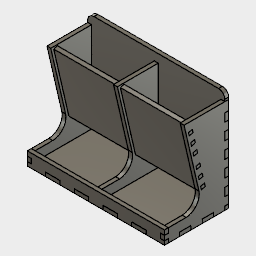
battery_box_v4 (Autodesk Fusion 360 design; units mm, degrees)
Autodesk Fusion 360 part; units mm, degrees
(part 1 of 2)
sketch "Sketch1" plane through (0, 0, 0) normal (0, 1, 0) x (1, 0, 0) in component "battery_box"
  line L0 (2.54, -2.54) -> (113.665, -2.54)
  line L1 (113.665, -2.54) -> (113.665, -54.61)
  line L2 (113.665, -54.61) -> (2.54, -54.61)
  line L3 (2.54, -54.61) -> (2.54, -2.54)
  line L4 (2.54, -2.54) -> (113.665, -2.54)
  line L5 (113.665, -2.54) -> (113.665, -5.715)
  line L6 (113.665, -5.715) -> (2.54, -5.715)
  line L7 (2.54, -5.715) -> (2.54, -2.54)
  line L8 (2.54, -2.54) -> (5.715, -2.54)
  line L9 (5.715, -2.54) -> (5.715, -54.61)
  line L10 (5.715, -54.61) -> (2.54, -54.61)
  line L11 (2.54, -54.61) -> (2.54, -2.54)
  line L12 (113.665, -2.54) -> (110.49, -2.54)
  line L13 (110.49, -2.54) -> (110.49, -54.61)
  line L14 (110.49, -54.61) -> (113.665, -54.61)
  line L15 (113.665, -54.61) -> (113.665, -2.54)
  line L16 (2.54, -54.61) -> (113.665, -54.61)
  line L17 (113.665, -54.61) -> (113.665, -51.435)
  line L18 (113.665, -51.435) -> (2.54, -51.435)
  line L19 (2.54, -51.435) -> (2.54, -54.61)
  line L20 (58.1025, -54.61) -> (56.515, -54.61)
  line L21 (56.515, -54.61) -> (56.515, -2.54) construction
  line L22 (56.515, -2.54) -> (58.1025, -2.54)
  line L23 (56.515, -2.54) -> (59.69, -2.54)
  line L24 (59.69, -2.54) -> (59.69, -54.61) construction
  line L25 (59.69, -54.61) -> (56.515, -54.61) construction
  line L26 (2.54, -20.955) -> (113.665, -20.955) construction
  line L27 (113.665, -20.955) -> (113.665, -24.13)
  line L28 (113.665, -24.13) -> (2.54, -24.13) construction
  line L29 (2.54, -24.13) -> (2.54, -20.955)
  line L30 (5.715, -5.715) -> (5.715, -2.54)
  dimension "d4" = 52.07
  dimension "d5" = 111.125
  dimension "d6" = 3.175
  dimension "d9" = 3.175
  dimension "d11" = 3.175
  dimension "d13" = 3.175
  dimension "d16" = 3.175
  dimension "d18" = 3.175
  dimension "d19" = 15.24
  measures "d4" distance of L0.start L2.end
  measures "d5" distance of L0.start L0.end
  measures "d6" distance of L0.start L6.end
  measures "d9" distance of L0.start L8.end
  measures "d11" distance of L0.end L12.end
  measures "d13" distance of L2.end L18.end
  measures "d16" distance of L21.end L23.end
  measures "d18" distance of L26.start L28.end
  measures "d19" distance of L6 L26
extrude "Extrude4" add sketch "Sketch1" against normal blind 3.175 makes body 1 in component "battery_box"
extrude "Extrude5" add sketch "Sketch1" along normal blind 7.62 separate body contours L2 L9 L13 L16 L18 L20 | L2 L3 L9 L10 L11 L16 L18 L19 | L1 L2 L13 L14 L15 L16 L17 L18 makes body 2 in component "battery_box"
extrude "Extrude6" add sketch "Sketch1" along normal blind 57.15 separate body contours L0 L3 L4 L6 L7 L8 L9 L11 L30 | L0 L4 L6 L9 L13 L22 L23 L30 | L0 L1 L4 L5 L6 L12 L13 L15 makes body 3 in component "battery_box"
extrude "Extrude7" add sketch "Sketch1" along normal blind 7.62 separate body contours L1 L6 L13 L15 L18 L27 makes body 4 in component "battery_box"
sketch "Side" plane through (113.665, 0, 0) normal (1, 0, 0) x (0, 0, -1) in component "battery_box"
  line L0 (-51.435, 0) -> (-5.715, 0)
  line L1 (-5.715, 0) -> (-5.715, 7.62)
  line L2 (-5.715, 7.62) -> (-51.435, 7.62)
  line L3 (-51.435, 7.62) -> (-51.435, 0)
  line L4 (-32.385, 45.72) -> (-5.715, 45.72)
  line L5 (-5.715, 45.72) -> (-5.715, 7.62)
  line L6 (-5.715, 7.62) -> (-20.955, 7.62)
  line L7 (-20.955, 7.62) -> (-20.955, 45.72)
  line L8 (-20.955, 45.72) -> (-5.715, 45.72)
  line L9 (-5.715, 45.72) -> (-5.715, 7.62)
  line L10 (-20.955, 7.62) -> (-24.13, 7.62)
  line L11 (-24.13, 45.72) -> (-20.955, 45.72)
  line L12 (-20.955, 45.72) -> (-20.955, 7.62)
  line L13 (-32.385, 45.72) -> (-26.6739, 20.9756)
  arc A0 (-37.0642, 7.62) -> (-26.6739, 20.9756) centre (-37.61, 18.7642) ccw
  line L14 (-5.715, 45.72) -> (-2.54, 45.72)
  line L15 (-2.54, 45.72) -> (-2.54, 0)
  line L16 (-2.54, -3.175) -> (-5.715, -3.175)
  line L17 (-5.715, 0) -> (-5.715, 45.72)
  line L18 (-51.435, 7.62) -> (-54.61, 7.62)
  line L19 (-54.61, 7.62) -> (-54.61, 0)
  line L20 (-54.61, 0) -> (-51.435, 0)
  line L21 (-51.435, 0) -> (-51.435, 7.62)
  line L22 (-54.61, 0) -> (-51.435, 0)
  line L23 (-51.435, 0) -> (-51.435, 3.81)
  line L24 (-51.435, 3.81) -> (-54.61, 3.81)
  line L25 (-54.61, 3.81) -> (-54.61, 0)
  line L26 (-5.715, 0) -> (-2.54, 0)
  line L27 (-2.54, 0) -> (-2.54, 45.72)
  line L28 (-2.54, 45.72) -> (-5.715, 45.72)
  line L29 (-5.715, 45.72) -> (-5.715, 0)
  line L30 (-5.715, 45.72) -> (-2.54, 45.72)
  line L31 (-5.715, 39.1886) -> (-2.54, 39.1886)
  line L32 (-5.715, 32.6571) -> (-2.54, 32.6571)
  line L33 (-5.715, 26.1257) -> (-2.54, 26.1257)
  line L34 (-5.715, 19.5943) -> (-2.54, 19.5943)
  line L35 (-5.715, 13.0629) -> (-2.54, 13.0629)
  line L36 (-5.715, 6.5314) -> (-2.54, 6.5314)
  line L37 (-5.715, 0) -> (-2.54, 0)
  line L38 (-51.435, 0) -> (-5.715, 0)
  line L39 (-5.715, 0) -> (-5.715, -3.175)
  line L40 (-5.715, -3.175) -> (-51.435, -3.175)
  line L41 (-51.435, -3.175) -> (-51.435, 0)
  line L42 (-51.435, 0) -> (-51.435, -3.175)
  line L43 (-42.291, 0) -> (-42.291, -3.175)
  line L44 (-33.147, 0) -> (-33.147, -3.175)
  line L45 (-24.003, 0) -> (-24.003, -3.175)
  line L46 (-14.859, 0) -> (-14.859, -3.175)
  line L47 (-5.715, 0) -> (-5.715, -3.175)
  point P0 (-2.54, -3.175)
  point P1 (-54.61, 0)
  point P2 (-54.61, 0)
  dimension "d34" = 45.72
  dimension "d36" = 15.24
  dimension "d37" = 38.1
  dimension "d38" = 3.175
  dimension "d39" = 38.1
  dimension "d42" = 0
  dimension "d43" = -45.72
  dimension "d46" = 45.72
  dimension "d47" = 0
  measures "d34" distance of L0.end L4.end
  measures "d36" distance of L1.end L6.end
  measures "d37" distance of L1.end L4.end
  measures "d38" distance of L6.end L10.end
  measures "d39" distance of L6.end L7.end
delete_body "RemoveBody1" bodies 4 in component "battery_box"
extrude "Extrude8" cut sketch "Side" against normal blind 3.175 contours L0 L1 L2 L3 L6 L10 L17 L21 L23 L29 L38 | L3 L19 L20 L21 L22 L23 L24 L25 | L0 L38 L40 L41 L42 L43 | L0 L38 L40 L44 L45 | L2 L4 L7 L10 L11 L12 L13 A0 | L0 L38 L39 L40 L46 L47 | L1 L15 L17 L26 L27 L29 L36 L37 | L2 L4 L5 L6 L7 L8 L9 L12 L17 L29 | L5 L9 L15 L17 L27 L29 L34 L35 | L5 L9 L14 L15 L17 L27 L28 L29 L30 L31 | L5 L9 L15 L17 L27 L29 L32 L33 bodies 1 2 3 in component "battery_box"
extrude "Extrude9" add sketch "Side" against normal blind 3.175 separate body contours L0 L1 L2 L3 L6 L10 L17 L21 L23 L29 L38 | L3 L19 L20 L21 L22 L23 L24 L25 | L0 L38 L40 L41 L42 L43 | L0 L38 L40 L44 L45 | L2 L4 L7 L10 L11 L12 L13 A0 | L0 L38 L39 L40 L46 L47 | L1 L15 L17 L26 L27 L29 L36 L37 | L2 L4 L5 L6 L7 L8 L9 L12 L17 L29 | L5 L9 L15 L17 L27 L29 L34 L35 | L5 L9 L14 L15 L17 L27 L28 L29 L30 L31 | L5 L9 L15 L17 L27 L29 L32 L33 makes body 5 in component "battery_box"
combine "Combine1" operation cut target body 3 tool bodies 5 keep tools in component "battery_box"
combine "Combine2" operation cut target body 1 tool bodies 5 keep tools in component "battery_box"
combine "Combine3" operation cut target body 2 tool bodies 5 keep tools in component "battery_box"
copy_body "CopyPasteBodies1" bodies 5 makes body 6 in component "battery_box"
move_body "Move1" bodies 6 to x (1, 0, 0) y (0, 1, 0) z (0, 0, 1) at (-107.95, 0, 0) in component "battery_box"
copy_body "CopyPasteBodies2" bodies 5 makes body 7 in component "battery_box"
move_body "Move2" bodies 7 to x (1, 0, 0) y (0, 1, 0) z (0, 0, 1) at (-53.975, 0, 0) in component "battery_box"
combine "Combine4" operation cut target body 3 tool bodies 7 6 keep tools in component "battery_box"
combine "Combine5" operation cut target body 1 tool bodies 6 7 keep tools in component "battery_box"
sketch "Sketch5" plane through (0, 0, 0) normal (0, 1, 0) x (-1, 0, 0) in component "battery_box"
sketch "Sketch6" plane through (0, 0, 54.61) normal (0, 0, 1) x (1, 0, 0) in component "battery_box"
  line L0 (110.49, 3.81) -> (113.665, 3.81)
  line L1 (113.665, 3.81) -> (113.665, 7.62)
  line L2 (113.665, 7.62) -> (2.54, 7.62)
  line L3 (2.54, 7.62) -> (2.54, 0)
  line L4 (2.54, 0) -> (110.49, 0)
  line L5 (110.49, 0) -> (110.49, 3.81)
  line L6 (5.715, 0) -> (110.49, 0)
  line L7 (110.49, 0) -> (110.49, -3.175)
  line L8 (110.49, -3.175) -> (5.715, -3.175)
  line L9 (5.715, -3.175) -> (5.715, 0)
  line L10 (5.715, 0) -> (5.715, -3.175)
  line L11 (17.3567, -3.175) -> (17.3567, 0)
  line L12 (28.9983, -3.175) -> (28.9983, 0)
  line L13 (40.64, -3.175) -> (40.64, 0)
  line L14 (52.2817, -3.175) -> (52.2817, 0)
  line L15 (63.9233, -3.175) -> (63.9233, 0)
  line L16 (75.565, -3.175) -> (75.565, 0)
  line L17 (87.2067, -3.175) -> (87.2067, 0)
  line L18 (98.8483, -3.175) -> (98.8483, 0)
  line L19 (110.49, -3.175) -> (110.49, 0)
  line L20 (2.54, 0) -> (113.665, 0)
  line L21 (113.665, 0) -> (113.665, -3.175)
  line L22 (113.665, -3.175) -> (2.54, -3.175)
  line L23 (2.54, -3.175) -> (2.54, 0)
  point P0 (5.715, 0)
  point P1 (113.665, -3.175)
  dimension "d62" = 104.775
  dimension "d63" = 3.175
  dimension "d66" = 104.775
  dimension "d67" = 0
  measures "d62" distance of P0 L4.end
  measures "d63" distance of P0 L8.end
extrude "Extrude10" add sketch "Sketch6" against normal blind 3.175 separate body contours L4 L6 L7 L8 L18 L19 L20 L22 | L7 L19 L20 L21 L22 | L4 L6 L8 L16 L17 L20 L22 | L4 L9 L10 L20 L22 L23 | L4 L6 L8 L9 L10 L11 L20 L22 | L4 L6 L8 L14 L15 L20 L22 | L4 L6 L8 L12 L13 L20 L22 makes body 8 at (83.3261, -3.175, 53.5517) makes body 9 at (60.0428, -3.175, 53.5517) makes body 10 at (108.7261, -3.175, 53.5517) makes body 11 at (32.8789, 0, 53.5517) makes body 12 at (7.4789, 0, 53.5517) in component "battery_box"
combine "Combine6" operation add target body 2 tool bodies 12 11 10 9 8 in component "battery_box"
combine "Combine7" operation cut target body 1 tool bodies 2 keep tools in component "battery_box"
combine "Combine8" operation cut target body 2 tool bodies 6 keep tools in component "battery_box"
sketch "Sketch7" plane through (0, -3.175, 0) normal (0, -1, 0) x (1, 0, 0) in component "battery_box"
  line L0 (59.69, 5.715) -> (56.515, 5.715)
  line L1 (56.515, 5.715) -> (56.515, 14.859)
  line L2 (56.515, 14.859) -> (59.69, 14.859)
  line L3 (59.69, 14.859) -> (59.69, 5.715)
  line L4 (59.69, 24.003) -> (56.515, 24.003)
  line L5 (56.515, 24.003) -> (56.515, 33.147)
  line L6 (56.515, 33.147) -> (59.69, 33.147)
  line L7 (59.69, 33.147) -> (59.69, 24.003)
  line L8 (110.49, 51.435) -> (98.8483, 51.435)
  line L9 (98.8483, 51.435) -> (98.8483, 54.61)
  line L10 (98.8483, 54.61) -> (87.2067, 54.61)
  line L11 (87.2067, 54.61) -> (87.2067, 51.435)
  line L12 (87.2067, 51.435) -> (75.565, 51.435)
  line L13 (75.565, 51.435) -> (75.565, 54.61)
  line L14 (75.565, 54.61) -> (63.9233, 54.61)
  line L15 (63.9233, 54.61) -> (63.9233, 51.435)
  line L16 (63.9233, 51.435) -> (59.69, 51.435)
  line L17 (59.69, 51.435) -> (59.69, 42.291)
  line L18 (59.69, 42.291) -> (56.515, 42.291)
  line L19 (56.515, 42.291) -> (56.515, 51.435)
  line L20 (56.515, 51.435) -> (52.2817, 51.435)
  line L21 (52.2817, 51.435) -> (52.2817, 54.61)
  line L22 (52.2817, 54.61) -> (40.64, 54.61)
  line L23 (40.64, 54.61) -> (40.64, 51.435)
  line L24 (40.64, 51.435) -> (28.9983, 51.435)
  line L25 (28.9983, 51.435) -> (28.9983, 54.61)
  line L26 (28.9983, 54.61) -> (17.3567, 54.61)
  line L27 (17.3567, 54.61) -> (17.3567, 51.435)
  line L28 (17.3567, 51.435) -> (5.715, 51.435)
  line L29 (5.715, 51.435) -> (5.715, 42.291)
  line L30 (5.715, 42.291) -> (2.54, 42.291)
  line L31 (2.54, 42.291) -> (2.54, 33.147)
  line L32 (2.54, 33.147) -> (5.715, 33.147)
  line L33 (5.715, 33.147) -> (5.715, 24.003)
  line L34 (5.715, 24.003) -> (2.54, 24.003)
  line L35 (2.54, 24.003) -> (2.54, 14.859)
  line L36 (2.54, 14.859) -> (5.715, 14.859)
  line L37 (5.715, 14.859) -> (5.715, 5.715)
  line L38 (5.715, 5.715) -> (2.54, 5.715)
  line L39 (2.54, 5.715) -> (2.54, 2.54)
  line L40 (2.54, 2.54) -> (113.665, 2.54)
  line L41 (113.665, 2.54) -> (113.665, 5.715)
  line L42 (113.665, 5.715) -> (110.49, 5.715)
  line L43 (110.49, 5.715) -> (110.49, 14.859)
  line L44 (110.49, 14.859) -> (113.665, 14.859)
  line L45 (113.665, 14.859) -> (113.665, 24.003)
  line L46 (113.665, 24.003) -> (110.49, 24.003)
  line L47 (110.49, 24.003) -> (110.49, 33.147)
  line L48 (110.49, 33.147) -> (113.665, 33.147)
  line L49 (113.665, 33.147) -> (113.665, 42.291)
  line L50 (113.665, 42.291) -> (110.49, 42.291)
  line L51 (110.49, 42.291) -> (110.49, 51.435)
  line L52 (2.54, 5.715) -> (113.665, 5.715)
  line L53 (113.665, 5.715) -> (113.665, 2.54)
  line L54 (113.665, 2.54) -> (2.54, 2.54)
  line L55 (2.54, 2.54) -> (2.54, 5.715)
  line L56 (2.54, 54.61) -> (17.3567, 54.61)
  line L57 (17.3567, 54.61) -> (17.3567, 51.435)
  line L58 (17.3567, 51.435) -> (2.54, 51.435)
  line L59 (2.54, 51.435) -> (2.54, 54.61)
  line L60 (28.9983, 54.61) -> (40.64, 54.61)
  line L61 (40.64, 54.61) -> (40.64, 51.435)
  line L62 (40.64, 51.435) -> (28.9983, 51.435)
  line L63 (28.9983, 51.435) -> (28.9983, 54.61)
  line L64 (52.2817, 54.61) -> (63.9233, 54.61)
  line L65 (63.9233, 54.61) -> (63.9233, 51.435)
  line L66 (63.9233, 51.435) -> (52.2817, 51.435)
  line L67 (52.2817, 51.435) -> (52.2817, 54.61)
  line L68 (75.565, 54.61) -> (87.2067, 54.61)
  line L69 (87.2067, 54.61) -> (87.2067, 51.435)
  line L70 (87.2067, 51.435) -> (75.565, 51.435)
  line L71 (75.565, 51.435) -> (75.565, 54.61)
  line L72 (98.8483, 54.61) -> (113.665, 54.61)
  line L73 (113.665, 54.61) -> (113.665, 51.435)
  line L74 (113.665, 51.435) -> (98.8483, 51.435)
  line L75 (98.8483, 51.435) -> (98.8483, 54.61)
  line L76 (2.54, 24.003) -> (2.54, 33.147)
  line L77 (113.665, 24.003) -> (113.665, 33.147)
  line L78 (2.54, 28.575) -> (113.665, 28.575) construction
  line L79 (17.3567, 2.54) -> (17.3567, 5.715)
  line L80 (40.64, 2.54) -> (40.64, 5.715)
  line L81 (28.9983, 5.715) -> (28.9983, 2.54)
  line L82 (52.2817, 5.715) -> (52.2817, 2.54)
  line L83 (63.9233, 5.715) -> (52.2817, 5.715)
  line L84 (63.9233, 2.54) -> (63.9233, 5.715)
  line L85 (75.565, 5.715) -> (75.565, 2.54)
  line L86 (87.2067, 5.715) -> (75.565, 5.715)
  line L87 (87.2067, 2.54) -> (87.2067, 5.715)
  line L88 (98.8483, 5.715) -> (98.8483, 2.54)
  line L89 (113.665, 5.715) -> (98.8483, 5.715)
  line L90 (113.665, 2.54) -> (113.665, 5.715)
  line L91 (98.8483, 2.54) -> (113.665, 2.54)
  line L92 (75.565, 2.54) -> (87.2067, 2.54)
  line L93 (52.2817, 2.54) -> (63.9233, 2.54)
  line L94 (28.9983, 2.54) -> (40.64, 2.54)
  line L95 (40.64, 5.715) -> (28.9983, 5.715)
  line L96 (2.54, 2.54) -> (17.3567, 2.54)
  line L97 (17.3567, 5.715) -> (2.54, 5.715)
  line L98 (2.54, 5.715) -> (2.54, 2.54)
  point P0 (2.54, 54.61)
  point P1 (113.665, 51.435)
extrude "Extrude11" add sketch "Sketch7" against normal blind 3.175 separate body contours L0 L40 L52 L54 L82 L83 L84 L93 | L40 L52 L54 L85 L86 L87 L92 | L40 L52 L54 L80 L81 L94 L95 | L40 L41 L42 L52 L53 L54 L88 L89 L90 L91 | L38 L39 L40 L52 L54 L55 L79 L96 L97 L98 makes body 13 at (56.1622, -2.1167, 2.54) makes body 14 at (32.8789, -2.1167, 5.715) makes body 15 at (79.4456, -2.1167, 5.715) makes body 16 at (7.4789, -1.0583, 5.715) makes body 17 at (108.7261, -1.0583, 5.715) in component "battery_box"
combine "Combine9" operation cut target body 1 tool bodies 13 14 15 16 17 keep tools in component "battery_box"
combine "Combine10" operation add target body 3 tool bodies 17 15 13 14 16 in component "battery_box"
sketch "Ramp" plane through (0, -4.7842, 20.7284) normal (0, -0.224893, 0.974384) x (1, 0, 0) in component "battery_box"
  line L0 (2.54, 0) -> (2.54, 18.415) construction
  line L1 (2.54, 18.415) -> (113.665, 18.415) construction
  line L2 (113.665, 18.415) -> (113.665, 0) construction
  line L3 (113.665, 18.415) -> (2.54, 18.415)
  line L4 (2.54, 18.415) -> (2.54, 45.72)
  line L5 (2.54, 45.72) -> (113.665, 45.72)
  line L6 (113.665, 45.72) -> (113.665, 18.415)
  line L7 (58.1025, 45.72) -> (58.1025, 18.415) construction
  line L8 (113.665, 45.72) -> (110.49, 45.72)
  line L9 (110.49, 45.72) -> (110.49, 18.415)
  line L10 (110.49, 18.415) -> (113.665, 18.415)
  line L11 (113.665, 18.415) -> (113.665, 45.72)
  line L12 (59.69, 45.72) -> (56.515, 45.72)
  line L13 (56.515, 45.72) -> (56.515, 18.415)
  line L14 (56.515, 18.415) -> (59.69, 18.415)
  line L15 (59.69, 18.415) -> (59.69, 45.72)
  line L16 (113.665, 45.72) -> (110.49, 45.72)
  line L17 (113.665, 45.72) -> (110.49, 45.72)
  line L18 (113.665, 45.72) -> (110.49, 45.72)
  line L19 (113.665, 18.415) -> (110.49, 18.415)
  line L20 (113.665, 18.415) -> (110.49, 18.415)
  line L21 (113.665, 18.415) -> (110.49, 18.415)
  line L22 (110.49, 18.415) -> (110.49, 45.72)
  line L23 (110.49, 45.72) -> (113.665, 45.72)
  line L24 (113.665, 45.72) -> (113.665, 18.415)
  line L25 (110.49, 21.1455) -> (113.665, 21.1455)
  line L26 (110.49, 23.876) -> (113.665, 23.876)
  line L27 (110.49, 26.6065) -> (113.665, 26.6065)
  line L28 (110.49, 29.337) -> (113.665, 29.337)
  line L29 (110.49, 32.0675) -> (113.665, 32.0675)
  line L30 (110.49, 34.798) -> (113.665, 34.798)
  line L31 (110.49, 37.5285) -> (113.665, 37.5285)
  line L32 (110.49, 40.259) -> (113.665, 40.259)
  line L33 (110.49, 42.9895) -> (113.665, 42.9895)
  line L34 (110.49, 45.72) -> (113.665, 45.72)
  line L35 (113.665, 18.415) -> (56.515, 18.415)
  line L36 (56.515, 18.415) -> (56.515, 45.72)
  line L37 (56.515, 45.72) -> (113.665, 45.72)
  line L38 (113.665, 45.72) -> (113.665, 18.415)
  line L39 (113.665, 18.415) -> (56.515, 18.415)
  line L40 (56.515, 18.415) -> (56.515, 45.72)
  line L41 (56.515, 45.72) -> (113.665, 45.72)
  line L42 (113.665, 45.72) -> (113.665, 18.415)
  line L43 (85.09, 18.415) -> (85.09, 45.72) construction
  line L44 (56.515, 45.72) -> (56.515, 18.415)
  line L45 (59.69, 18.415) -> (59.69, 45.72)
  line L46 (56.515, 18.415) -> (56.515, 45.72)
  line L47 (59.69, 45.72) -> (59.69, 18.415)
  line L48 (56.515, 45.72) -> (56.515, 18.415)
  line L49 (56.515, 45.72) -> (56.515, 18.415)
  line L50 (56.515, 45.72) -> (56.515, 18.415)
  line L51 (59.69, 26.6065) -> (56.515, 26.6065)
  line L52 (59.69, 29.337) -> (56.515, 29.337)
  line L53 (59.69, 23.876) -> (56.515, 23.876)
  line L54 (59.69, 45.72) -> (56.515, 45.72)
  line L55 (59.69, 37.5285) -> (56.515, 37.5285)
  line L56 (59.69, 40.259) -> (56.515, 40.259)
  line L57 (59.69, 42.9895) -> (56.515, 42.9895)
  line L58 (59.69, 45.72) -> (56.515, 45.72)
  line L59 (59.69, 34.798) -> (56.515, 34.798)
  line L60 (59.69, 21.1455) -> (56.515, 21.1455)
  line L61 (59.69, 32.0675) -> (56.515, 32.0675)
  line L62 (56.515, 45.72) -> (59.69, 45.72)
  line L63 (56.515, 45.72) -> (59.69, 45.72)
  line L64 (56.515, 18.415) -> (59.69, 18.415)
  line L65 (56.515, 18.415) -> (59.69, 18.415)
  line L66 (56.515, 45.72) -> (59.69, 45.72)
  line L67 (59.69, 18.415) -> (56.515, 18.415)
  line L68 (56.515, 18.415) -> (59.69, 18.415)
  line L69 (56.515, 45.72) -> (59.69, 45.72)
  line L70 (2.54, 45.72) -> (2.54, 18.415)
  line L71 (5.715, 45.72) -> (2.54, 45.72)
  line L72 (2.54, 45.72) -> (2.54, 18.415)
  line L73 (5.715, 45.72) -> (5.715, 18.415)
  line L74 (5.715, 18.415) -> (2.54, 18.415)
  line L75 (2.54, 18.415) -> (2.54, 45.72)
  line L76 (2.54, 45.72) -> (5.715, 45.72)
  line L77 (2.54, 45.72) -> (5.715, 45.72)
  line L78 (2.54, 45.72) -> (5.715, 45.72)
  line L79 (2.54, 45.72) -> (2.54, 18.415)
  line L80 (5.715, 21.1455) -> (2.54, 21.1455)
  line L81 (5.715, 26.6065) -> (2.54, 26.6065)
  line L82 (2.54, 18.415) -> (5.715, 18.415)
  line L83 (2.54, 18.415) -> (5.715, 18.415)
  line L84 (5.715, 18.415) -> (5.715, 45.72)
  line L85 (2.54, 45.72) -> (2.54, 18.415)
  line L86 (5.715, 23.876) -> (2.54, 23.876)
  line L87 (5.715, 32.0675) -> (2.54, 32.0675)
  line L88 (2.54, 45.72) -> (5.715, 45.72)
  line L89 (5.715, 34.798) -> (2.54, 34.798)
  line L90 (5.715, 45.72) -> (2.54, 45.72)
  line L91 (2.54, 18.415) -> (5.715, 18.415)
  line L92 (5.715, 37.5285) -> (2.54, 37.5285)
  line L93 (5.715, 40.259) -> (2.54, 40.259)
  line L94 (5.715, 42.9895) -> (2.54, 42.9895)
  line L95 (5.715, 29.337) -> (2.54, 29.337)
  line L96 (56.515, 26.437) -> (59.69, 26.437)
  point P0 (2.54, 45.72)
  point P1 (59.69, 45.72)
  dimension "d77" = 111.125
  dimension "d79" = 27.305
  dimension "d80" = 3.175
  dimension "d81" = 27.305
  dimension "d85" = 0
  dimension "d86" = 27.305
  measures "d77" distance of L2.end L0.start
  measures "d79" distance of L5.end L1.end
  measures "d80" distance of L5.end L8.end
  measures "d81" distance of P1 L14.end
extrude "Extrude12" add sketch "Ramp" against normal blind 3.175 separate body contours L3 L5 L13 L36 L40 L44 L46 L48 L49 L50 L73 L84 | L13 L15 L36 L40 L44 L45 L46 L47 L48 L49 L50 L53 L96 | L4 L70 L72 L73 L75 L79 L81 L84 L85 L86 | L13 L15 L36 L40 L44 L45 L46 L47 L48 L49 L50 L59 L61 | L4 L70 L72 L73 L75 L79 L84 L85 L87 L89 | L13 L15 L36 L40 L44 L45 L46 L47 L48 L49 L50 L56 L57 | L4 L70 L72 L73 L75 L79 L84 L85 L93 L94 makes body 18 in component "battery_box"
move_body "Move3" bodies 18 to x (1, 0, 0) y (0, 1, 0) z (0, 0, 1) at (0, 0, -3.175) in component "battery_box"
move_body "Move4" bodies 18 to x (1, 0, 0) y (0, 1, 0) z (0, 0, 1) at (0, 5.08, 2.413) in component "battery_box"
copy_body "CopyPasteBodies3" bodies 18 makes body 19 in component "battery_box"
move_body "Move5" bodies 19 to x (1, 0, 0) y (0, 1, 0) z (0, 0, 1) at (53.975, 0, 0) in component "battery_box"
move_body "Move6" bodies 19 to x (1, 0, 0) y (0, -1, 0) z (0, 0, -1) at (0, 36.4781, 42.0282) in component "battery_box"
move_body "Align1" bodies 19 to x (1, 0, 0) y (0, 1, 0) z (0, 0, 1) at (0, 27.3196, 9.2344) in component "battery_box"
combine "Combine11" operation cut target body 5 tool bodies 19 keep tools in component "battery_box"
combine "Combine12" operation cut target body 6 tool bodies 18 keep tools in component "battery_box"
combine "Combine13" operation cut target body 7 tool bodies 19 18 keep tools in component "battery_box"
sketch "Sketch10" plane through (59.69, 0, 0) normal (1, 0, 0) x (0, 0, -1) in component "battery_box"
  line L0 (-2.54, 0) -> (-2.54, 6.5314)
  line L1 (-2.54, 6.5314) -> (-5.715, 6.5314)
  line L2 (-5.715, 6.5314) -> (-5.715, 13.0629)
  line L3 (-5.715, 13.0629) -> (-2.54, 13.0629)
  line L4 (-2.54, 13.0629) -> (-2.54, 19.5943)
  line L5 (-2.54, 19.5943) -> (-5.715, 19.5943)
  line L6 (-5.715, 19.5943) -> (-5.715, 26.1257)
  line L7 (-5.715, 26.1257) -> (-2.54, 26.1257)
  line L8 (-2.54, 26.1257) -> (-2.54, 32.6571)
  line L9 (-2.54, 32.6571) -> (-5.715, 32.6571)
  line L10 (-5.715, 32.6571) -> (-5.715, 39.1886)
  line L11 (-5.715, 39.1886) -> (-2.54, 39.1886)
  line L12 (-2.54, 39.1886) -> (-2.54, 45.72)
  line L13 (-2.54, 45.72) -> (-32.385, 45.72)
  line L14 (-32.385, 45.72) -> (-26.6739, 20.9756)
  arc A0 (-37.0642, 7.62) -> (-26.6739, 20.9756) centre (-37.61, 18.7642) ccw
  line L15 (-37.0642, 7.62) -> (-51.435, 7.62)
  line L16 (-51.435, 7.62) -> (-51.435, 3.81)
  line L17 (-51.435, 3.81) -> (-54.61, 3.81)
  line L18 (-54.61, 3.81) -> (-54.61, 0)
  line L19 (-54.61, 0) -> (-51.435, 0)
  line L20 (-51.435, 0) -> (-51.435, -3.175)
  line L21 (-51.435, -3.175) -> (-42.291, -3.175)
  line L22 (-42.291, -3.175) -> (-42.291, 0)
  line L23 (-42.291, 0) -> (-33.147, 0)
  line L24 (-33.147, 0) -> (-33.147, -3.175)
  line L25 (-33.147, -3.175) -> (-24.003, -3.175)
  line L26 (-24.003, -3.175) -> (-24.003, 0)
  line L27 (-24.003, 0) -> (-14.859, 0)
  line L28 (-14.859, 0) -> (-14.859, -3.175)
  line L29 (-14.859, -3.175) -> (-5.715, -3.175)
  line L30 (-5.715, -3.175) -> (-5.715, 0)
  line L31 (-5.715, 0) -> (-2.54, 0)
  line L32 (-28.4063, 36.8629) -> (-29.6344, 42.184)
  line L33 (-29.6344, 42.184) -> (-26.5407, 42.8981)
  line L34 (-26.5407, 42.8981) -> (-25.3126, 37.577)
  line L35 (-25.3126, 37.577) -> (-28.4063, 36.8629)
  line L36 (-26.564, 28.8813) -> (-27.7922, 34.2024)
  line L37 (-27.7922, 34.2024) -> (-24.6985, 34.9164)
  line L38 (-24.6985, 34.9164) -> (-23.4704, 29.5953)
  line L39 (-23.4704, 29.5953) -> (-26.564, 28.8813)
  line L40 (-24.7218, 20.8996) -> (-25.9119, 26.0556)
  line L41 (-25.9119, 26.0556) -> (-22.8182, 26.7696)
  line L42 (-22.8182, 26.7696) -> (-21.6282, 21.6136)
  line L43 (-21.6282, 21.6136) -> (-24.7218, 20.8996)
  line L44 (-54.61, 3.81) -> (-51.435, 3.81)
  line L45 (-51.435, 3.81) -> (-51.435, 0)
  line L46 (-51.435, 0) -> (-54.61, 0)
  line L47 (-54.61, 0) -> (-54.61, 3.81)
extrude "Extrude13" cut sketch "Sketch10" against normal blind 3.175 contours L17 L18 L19 L44 L45 L46 L47 bodies 7 in component "battery_box"
copy_body "CopyPasteBodies4" bodies 18 makes body 20 in component "battery_box"
move_body "Move7" bodies 20 to x (1, 0, 0) y (0, 1, 0) z (0, 0, 1) at (0, 36.83, 0) in component "battery_box"
move_body "Align2" bodies 20 to x (1, 0, 0) y (0, 1, 0) z (0, 0, 1) at (0, -8.3617, -1.9299) in component "battery_box"
move_body "Align3" bodies 20 to x (1, 0, 0) y (0, 1, 0) z (0, 0, 1) at (0, -1.8627, 8.0706) in component "battery_box"
copy_body "CopyPasteBodies5" bodies 19 makes body 21 in component "battery_box"
move_body "Move8" bodies 21 to x (1, 0, 0) y (0, 1, 0) z (0, 0, 1) at (0, 38.1, 0) in component "battery_box"
move_body "Align4" bodies 21 to x (1, 0, 0) y (0, 1, 0) z (0, 0, 1) at (0, -11.4945, 6.1407) in component "battery_box"
combine "Combine14" operation add target body 21 tool bodies 19 in component "battery_box"
combine "Combine15" operation add target body 20 tool bodies 18 in component "battery_box"
sketch "Sketch11" plane through (113.665, 0, 0) normal (1, 0, 0) x (0, 0, -1) in component "battery_box"
  line L0 (-21.6282, 21.6136) -> (-24.7218, 20.8996)
  line L1 (-24.7218, 20.8996) -> (-25.3359, 23.5602)
  line L2 (-25.3359, 23.5602) -> (-22.2422, 24.2742)
  line L3 (-22.2422, 24.2742) -> (-21.6282, 21.6136)
  line L4 (-25.3507, 37.7421) -> (-28.4444, 37.0281)
  line L5 (-28.4444, 37.0281) -> (-29.0203, 39.5235)
  line L6 (-29.0203, 39.5235) -> (-25.9267, 40.2375)
  line L7 (-25.9267, 40.2375) -> (-25.3507, 37.7421)
  line L8 (-23.4704, 29.5953) -> (-26.564, 28.8813)
  line L9 (-26.564, 28.8813) -> (-27.1781, 31.5418)
  line L10 (-27.1781, 31.5418) -> (-24.0844, 32.2559)
  line L11 (-24.0844, 32.2559) -> (-23.4704, 29.5953)
  line L12 (-2.54, 0) -> (-2.54, 6.5314)
  line L13 (-2.54, 6.5314) -> (-5.715, 6.5314)
  line L14 (-5.715, 6.5314) -> (-5.715, 13.0629)
  line L15 (-5.715, 13.0629) -> (-2.54, 13.0629)
  line L16 (-2.54, 13.0629) -> (-2.54, 19.5943)
  line L17 (-2.54, 19.5943) -> (-5.715, 19.5943)
  line L18 (-5.715, 19.5943) -> (-5.715, 26.1257)
  line L19 (-5.715, 26.1257) -> (-2.54, 26.1257)
  line L20 (-2.54, 26.1257) -> (-2.54, 32.6571)
  line L21 (-2.54, 32.6571) -> (-5.715, 32.6571)
  line L22 (-5.715, 32.6571) -> (-5.715, 39.1886)
  line L23 (-5.715, 39.1886) -> (-2.54, 39.1886)
  line L24 (-2.54, 39.1886) -> (-2.54, 45.72)
  line L25 (-2.54, 45.72) -> (-32.385, 45.72)
  line L26 (-32.385, 45.72) -> (-26.6739, 20.9756)
  arc A0 (-37.0642, 7.62) -> (-26.6739, 20.9756) centre (-37.61, 18.7642) ccw
  line L27 (-37.0642, 7.62) -> (-51.435, 7.62)
  line L28 (-51.435, 7.62) -> (-51.435, 3.81)
  line L29 (-51.435, 3.81) -> (-54.61, 3.81)
  line L30 (-54.61, 3.81) -> (-54.61, 0)
  line L31 (-54.61, 0) -> (-51.435, 0)
  line L32 (-51.435, 0) -> (-51.435, -3.175)
  line L33 (-51.435, -3.175) -> (-42.291, -3.175)
  line L34 (-42.291, -3.175) -> (-42.291, 0)
  line L35 (-42.291, 0) -> (-33.147, 0)
  line L36 (-33.147, 0) -> (-33.147, -3.175)
  line L37 (-33.147, -3.175) -> (-24.003, -3.175)
  line L38 (-24.003, -3.175) -> (-24.003, 0)
  line L39 (-24.003, 0) -> (-14.859, 0)
  line L40 (-14.859, 0) -> (-14.859, -3.175)
  line L41 (-14.859, -3.175) -> (-5.715, -3.175)
  line L42 (-5.715, -3.175) -> (-5.715, 0)
  line L43 (-5.715, 0) -> (-2.54, 0)
  line L44 (-2.54, 45.72) -> (-32.385, 45.72)
  line L45 (-33.2955, 73.1704) -> (-2.54, 73.1704)
  line L46 (-2.54, 73.1704) -> (-2.54, 45.72)
  line L47 (-32.385, 45.72) -> (-39.0731, 74.6971)
  line L48 (-33.2955, 73.1704) -> (-38.7207, 73.1704)
extrude "Extrude14" add sketch "Sketch11" against normal blind 3.175 separate body contours L25 L44 L45 L46 L47 L48 makes body 22 in component "battery_box"
combine "Combine16" operation add target body 22 tool bodies 5 in component "battery_box"
delete_body "RemoveBody2" bodies 7 in component "battery_box"
delete_body "RemoveBody3" bodies 6 in component "battery_box"
sketch "Sketch12" plane through (113.665, 0, 0) normal (1, 0, 0) x (0, 0, -1) in component "battery_box"
  line L0 (-23.4704, 29.5953) -> (-26.564, 28.8813)
  line L1 (-26.564, 28.8813) -> (-27.1781, 31.5418)
  line L2 (-27.1781, 31.5418) -> (-24.0844, 32.2559)
  line L3 (-24.0844, 32.2559) -> (-23.4704, 29.5953)
  line L4 (-25.3507, 37.7421) -> (-28.4444, 37.0281)
  line L5 (-28.4444, 37.0281) -> (-29.0203, 39.5235)
  line L6 (-29.0203, 39.5235) -> (-25.9267, 40.2375)
  line L7 (-25.9267, 40.2375) -> (-25.3507, 37.7421)
  line L8 (-21.6282, 21.6136) -> (-24.7218, 20.8996)
  line L9 (-24.7218, 20.8996) -> (-25.3359, 23.5602)
  line L10 (-25.3359, 23.5602) -> (-22.2422, 24.2742)
  line L11 (-22.2422, 24.2742) -> (-21.6282, 21.6136)
  line L12 (-2.54, 73.1704) -> (-38.7207, 73.1704)
  line L13 (-38.7207, 73.1704) -> (-26.6739, 20.9756)
  arc A0 (-37.0642, 7.62) -> (-26.6739, 20.9756) centre (-37.61, 18.7642) ccw
  line L14 (-37.0642, 7.62) -> (-51.435, 7.62)
  line L15 (-51.435, 7.62) -> (-51.435, 3.81)
  line L16 (-51.435, 3.81) -> (-54.61, 3.81)
  line L17 (-54.61, 3.81) -> (-54.61, 0)
  line L18 (-54.61, 0) -> (-51.435, 0)
  line L19 (-51.435, 0) -> (-51.435, -3.175)
  line L20 (-51.435, -3.175) -> (-42.291, -3.175)
  line L21 (-42.291, -3.175) -> (-42.291, 0)
  line L22 (-42.291, 0) -> (-33.147, 0)
  line L23 (-33.147, 0) -> (-33.147, -3.175)
  line L24 (-33.147, -3.175) -> (-24.003, -3.175)
  line L25 (-24.003, -3.175) -> (-24.003, 0)
  line L26 (-24.003, 0) -> (-14.859, 0)
  line L27 (-14.859, 0) -> (-14.859, -3.175)
  line L28 (-14.859, -3.175) -> (-5.715, -3.175)
  line L29 (-5.715, -3.175) -> (-5.715, 0)
  line L30 (-5.715, 0) -> (-2.54, 0)
  line L31 (-2.54, 0) -> (-2.54, 6.5314)
  line L32 (-2.54, 6.5314) -> (-5.715, 6.5314)
  line L33 (-5.715, 6.5314) -> (-5.715, 13.0629)
  line L34 (-5.715, 13.0629) -> (-2.54, 13.0629)
  line L35 (-2.54, 13.0629) -> (-2.54, 19.5943)
  line L36 (-2.54, 19.5943) -> (-5.715, 19.5943)
  line L37 (-5.715, 19.5943) -> (-5.715, 26.1257)
  line L38 (-5.715, 26.1257) -> (-2.54, 26.1257)
  line L39 (-2.54, 26.1257) -> (-2.54, 32.6571)
  line L40 (-5.715, 32.6571) -> (-5.715, 39.1886)
  line L41 (-5.715, 39.1886) -> (-2.54, 39.1886)
  line L42 (-2.54, 39.1886) -> (-2.54, 73.1704)
  line L43 (-5.715, 13.0629) -> (-2.54, 13.0629)
  line L44 (-2.54, 13.0629) -> (-2.54, 6.5314)
  line L45 (-2.54, 6.5314) -> (-5.715, 6.5314)
  line L46 (-5.715, 6.5314) -> (-5.715, 13.0629)
  line L47 (-5.715, 26.1257) -> (-2.54, 26.1257)
  line L48 (-2.54, 26.1257) -> (-2.54, 19.5943)
  line L49 (-2.54, 19.5943) -> (-5.715, 19.5943)
  line L50 (-5.715, 19.5943) -> (-5.715, 26.1257)
  line L51 (-5.715, 32.6571) -> (-2.54, 32.6571)
  line L52 (-2.54, 45.72) -> (-5.715, 45.72)
  line L53 (-2.54, 39.1886) -> (-2.54, 45.72)
  line L54 (-5.715, 39.1886) -> (-2.54, 39.1886)
  line L55 (-5.715, 45.72) -> (-5.715, 39.1886)
  line L56 (-5.715, 52.2514) -> (-2.54, 52.2514)
  line L57 (-5.715, 58.7829) -> (-5.715, 52.2514)
  line L58 (-2.54, 52.2514) -> (-2.54, 58.7829)
  line L59 (-2.54, 58.7829) -> (-5.715, 58.7829)
  line L60 (-5.715, 52.2514) -> (-2.54, 52.2514)
  line L61 (-2.54, 52.2514) -> (-2.54, 45.72)
  line L62 (-2.54, 45.72) -> (-5.715, 45.72)
  line L63 (-5.715, 45.72) -> (-5.715, 52.2514)
  line L64 (-5.715, 58.7829) -> (-2.54, 58.7829)
  line L65 (-5.715, 65.3143) -> (-5.715, 58.7829)
  line L66 (-2.54, 58.7829) -> (-2.54, 65.3143)
  line L67 (-2.54, 65.3143) -> (-5.715, 65.3143)
  line L68 (-5.715, 62.0486) -> (-2.54, 62.0486)
  line L69 (-5.715, 58.7829) -> (-2.54, 58.7829)
  line L70 (-2.54, 58.7829) -> (-2.54, 52.2514)
  line L71 (-2.54, 52.2514) -> (-5.715, 52.2514)
  line L72 (-5.715, 52.2514) -> (-5.715, 58.7829)
  line L73 (-5.715, 71.8457) -> (-5.715, 65.3143)
  line L74 (-5.715, 65.3143) -> (-2.54, 65.3143)
  line L75 (-2.54, 65.3143) -> (-2.54, 71.8457)
  line L76 (-2.54, 71.8457) -> (-5.715, 71.8457)
extrude "Extrude15" add sketch "Sketch12" against normal blind 3.175 separate body contours L42 L65 L66 L67 L68 L74 | L42 L59 L64 L65 L66 L68 L69 | L42 L52 L56 L60 L61 L62 L63 L71 makes body 23 at (112.6067, 47.8971, 5.715) makes body 24 at (112.6067, 60.96, 2.54) in component "battery_box"
sketch "Sketch13" plane through (0, 0, 2.54) normal (0, 0, -1) x (-1, 0, 0) in component "battery_box"
  line L0 (-59.69, 0) -> (-59.69, 6.5314)
  line L1 (-59.69, 6.5314) -> (-56.515, 6.5314)
  line L2 (-56.515, 6.5314) -> (-56.515, 0)
  line L3 (-56.515, 0) -> (-59.69, 0)
  line L4 (-63.9233, 0) -> (-63.9233, -3.175)
  line L5 (-63.9233, -3.175) -> (-52.2817, -3.175)
  line L6 (-52.2817, -3.175) -> (-52.2817, 0)
  line L7 (-52.2817, 0) -> (-40.64, 0)
  line L8 (-40.64, 0) -> (-40.64, -3.175)
  line L9 (-40.64, -3.175) -> (-28.9983, -3.175)
  line L10 (-28.9983, -3.175) -> (-28.9983, 0)
  line L11 (-28.9983, 0) -> (-17.3567, 0)
  line L12 (-17.3567, 0) -> (-17.3567, -3.175)
  line L13 (-17.3567, -3.175) -> (-2.54, -3.175)
  line L14 (-2.54, -3.175) -> (-2.54, 0)
  line L15 (-2.54, 0) -> (-5.715, 0)
  line L16 (-5.715, 0) -> (-5.715, 6.5314)
  line L17 (-5.715, 6.5314) -> (-2.54, 6.5314)
  line L18 (-2.54, 6.5314) -> (-2.54, 13.0629)
  line L19 (-2.54, 13.0629) -> (-5.715, 13.0629)
  line L20 (-5.715, 13.0629) -> (-5.715, 19.5943)
  line L21 (-5.715, 19.5943) -> (-2.54, 19.5943)
  line L22 (-2.54, 19.5943) -> (-2.54, 26.1257)
  line L23 (-2.54, 26.1257) -> (-5.715, 26.1257)
  line L24 (-5.715, 26.1257) -> (-5.715, 32.6571)
  line L25 (-5.715, 32.6571) -> (-2.54, 32.6571)
  line L26 (-2.54, 32.6571) -> (-2.54, 39.1886)
  line L27 (-2.54, 39.1886) -> (-5.715, 39.1886)
  line L28 (-5.715, 39.1886) -> (-5.715, 45.72)
  line L29 (-5.715, 45.72) -> (-2.54, 45.72)
  line L30 (-2.54, 45.72) -> (-2.54, 57.15)
  line L31 (-2.54, 57.15) -> (-113.665, 57.15)
  line L32 (-113.665, 57.15) -> (-113.665, 45.72)
  line L33 (-113.665, 45.72) -> (-110.49, 45.72)
  line L34 (-110.49, 45.72) -> (-110.49, 39.1886)
  line L35 (-110.49, 39.1886) -> (-113.665, 39.1886)
  line L36 (-113.665, 39.1886) -> (-113.665, 32.6571)
  line L37 (-113.665, 32.6571) -> (-110.49, 32.6571)
  line L38 (-110.49, 32.6571) -> (-110.49, 26.1257)
  line L39 (-110.49, 26.1257) -> (-113.665, 26.1257)
  line L40 (-113.665, 26.1257) -> (-113.665, 19.5943)
  line L41 (-113.665, 19.5943) -> (-110.49, 19.5943)
  line L42 (-110.49, 19.5943) -> (-110.49, 13.0629)
  line L43 (-110.49, 13.0629) -> (-113.665, 13.0629)
  line L44 (-113.665, 13.0629) -> (-113.665, 6.5314)
  line L45 (-113.665, 6.5314) -> (-110.49, 6.5314)
  line L46 (-110.49, 6.5314) -> (-110.49, 0)
  line L47 (-110.49, 0) -> (-113.665, 0)
  line L48 (-113.665, 0) -> (-113.665, -3.175)
  line L49 (-113.665, -3.175) -> (-98.8483, -3.175)
  line L50 (-98.8483, -3.175) -> (-98.8483, 0)
  line L51 (-98.8483, 0) -> (-87.2067, 0)
  line L52 (-87.2067, 0) -> (-87.2067, -3.175)
  line L53 (-87.2067, -3.175) -> (-75.565, -3.175)
  line L54 (-75.565, -3.175) -> (-75.565, 0)
  line L55 (-75.565, 0) -> (-63.9233, 0)
  line L56 (-59.69, 45.72) -> (-56.515, 45.72)
  line L57 (-56.515, 45.72) -> (-56.515, 39.1886)
  line L58 (-56.515, 39.1886) -> (-59.69, 39.1886)
  line L59 (-59.69, 39.1886) -> (-59.69, 45.72)
  line L60 (-59.69, 32.6571) -> (-56.515, 32.6571)
  line L61 (-56.515, 32.6571) -> (-56.515, 26.1257)
  line L62 (-56.515, 26.1257) -> (-59.69, 26.1257)
  line L63 (-59.69, 26.1257) -> (-59.69, 32.6571)
  line L64 (-59.69, 19.5943) -> (-56.515, 19.5943)
  line L65 (-56.515, 19.5943) -> (-56.515, 13.0629)
  line L66 (-56.515, 13.0629) -> (-59.69, 13.0629)
  line L67 (-59.69, 13.0629) -> (-59.69, 19.5943)
  line L68 (-113.665, 57.15) -> (-2.54, 57.15)
  line L69 (-2.54, 57.15) -> (-2.54, 95.4786)
  line L70 (-2.54, 95.4786) -> (-113.665, 95.4786)
  line L71 (-113.665, 95.4786) -> (-113.665, 57.15)
  dimension "d131" = 111.125
  dimension "d132" = 38.3286
  measures "d131" distance of L31.end L30.end
  measures "d132" distance of L31.end L70.end
extrude "Extrude16" add sketch "Sketch13" against normal blind 3.175 separate body contours L31 L68 L69 L70 L71 makes body 25 in component "battery_box"
combine "Combine17" operation add target body 3 tool bodies 25 in component "battery_box"
combine "Combine18" operation cut target body 22 tool bodies 23 24 keep tools in component "battery_box"
combine "Combine19" operation cut target body 3 tool bodies 22 keep tools in component "battery_box"
delete_body "RemoveBody4" bodies 23 in component "battery_box"
delete_body "RemoveBody5" bodies 24 in component "battery_box"
sketch "Sketch14" plane through (0, 0, 2.54) normal (0, 0, -1) x (-1, 0, 0) in component "battery_box"
  line L0 (-59.69, 19.5943) -> (-56.515, 19.5943)
  line L1 (-56.515, 19.5943) -> (-56.515, 13.0629)
  line L2 (-56.515, 13.0629) -> (-59.69, 13.0629)
  line L3 (-59.69, 13.0629) -> (-59.69, 19.5943)
  line L4 (-59.69, 32.6571) -> (-56.515, 32.6571)
  line L5 (-56.515, 32.6571) -> (-56.515, 26.1257)
  line L6 (-56.515, 26.1257) -> (-59.69, 26.1257)
  line L7 (-59.69, 26.1257) -> (-59.69, 32.6571)
  line L8 (-59.69, 45.72) -> (-56.515, 45.72)
  line L9 (-56.515, 45.72) -> (-56.515, 39.1886)
  line L10 (-56.515, 39.1886) -> (-59.69, 39.1886)
  line L11 (-59.69, 39.1886) -> (-59.69, 45.72)
  line L12 (-113.665, 73.1704) -> (-110.49, 73.1704)
  line L13 (-110.49, 73.1704) -> (-110.49, 65.3143)
  line L14 (-110.49, 65.3143) -> (-113.665, 65.3143)
  line L15 (-113.665, 65.3143) -> (-113.665, 58.7829)
  line L16 (-113.665, 58.7829) -> (-110.49, 58.7829)
  line L17 (-110.49, 58.7829) -> (-110.49, 52.2514)
  line L18 (-110.49, 52.2514) -> (-113.665, 52.2514)
  line L19 (-113.665, 52.2514) -> (-113.665, 45.72)
  line L20 (-113.665, 45.72) -> (-110.49, 45.72)
  line L21 (-110.49, 45.72) -> (-110.49, 39.1886)
  line L22 (-110.49, 39.1886) -> (-113.665, 39.1886)
  line L23 (-113.665, 39.1886) -> (-113.665, 32.6571)
  line L24 (-113.665, 32.6571) -> (-110.49, 32.6571)
  line L25 (-110.49, 32.6571) -> (-110.49, 26.1257)
  line L26 (-110.49, 26.1257) -> (-113.665, 26.1257)
  line L27 (-113.665, 26.1257) -> (-113.665, 19.5943)
  line L28 (-113.665, 19.5943) -> (-110.49, 19.5943)
  line L29 (-110.49, 19.5943) -> (-110.49, 13.0629)
  line L30 (-110.49, 13.0629) -> (-113.665, 13.0629)
  line L31 (-113.665, 13.0629) -> (-113.665, 6.5314)
  line L32 (-113.665, 6.5314) -> (-110.49, 6.5314)
  line L33 (-110.49, 6.5314) -> (-110.49, 0)
  line L34 (-110.49, 0) -> (-113.665, 0)
  line L35 (-113.665, 0) -> (-113.665, -3.175)
  line L36 (-113.665, -3.175) -> (-98.8483, -3.175)
  line L37 (-98.8483, -3.175) -> (-98.8483, 0)
  line L38 (-98.8483, 0) -> (-87.2067, 0)
  line L39 (-87.2067, 0) -> (-87.2067, -3.175)
  line L40 (-87.2067, -3.175) -> (-75.565, -3.175)
  line L41 (-75.565, -3.175) -> (-75.565, 0)
  line L42 (-75.565, 0) -> (-63.9233, 0)
  line L43 (-63.9233, 0) -> (-63.9233, -3.175)
  line L44 (-63.9233, -3.175) -> (-52.2817, -3.175)
  line L45 (-52.2817, -3.175) -> (-52.2817, 0)
  line L46 (-52.2817, 0) -> (-40.64, 0)
  line L47 (-40.64, 0) -> (-40.64, -3.175)
  line L48 (-40.64, -3.175) -> (-28.9983, -3.175)
  line L49 (-28.9983, -3.175) -> (-28.9983, 0)
  line L50 (-28.9983, 0) -> (-17.3567, 0)
  line L51 (-17.3567, 0) -> (-17.3567, -3.175)
  line L52 (-17.3567, -3.175) -> (-2.54, -3.175)
  line L53 (-2.54, -3.175) -> (-2.54, 0)
  line L54 (-2.54, 0) -> (-5.715, 0)
  line L55 (-5.715, 0) -> (-5.715, 6.5314)
  line L56 (-5.715, 6.5314) -> (-2.54, 6.5314)
  line L57 (-2.54, 6.5314) -> (-2.54, 13.0629)
  line L58 (-2.54, 13.0629) -> (-5.715, 13.0629)
  line L59 (-5.715, 13.0629) -> (-5.715, 19.5943)
  line L60 (-5.715, 19.5943) -> (-2.54, 19.5943)
  line L61 (-2.54, 19.5943) -> (-2.54, 26.1257)
  line L62 (-2.54, 26.1257) -> (-5.715, 26.1257)
  line L63 (-5.715, 26.1257) -> (-5.715, 32.6571)
  line L64 (-5.715, 32.6571) -> (-2.54, 32.6571)
  line L65 (-2.54, 32.6571) -> (-2.54, 39.1886)
  line L66 (-2.54, 39.1886) -> (-5.715, 39.1886)
  line L67 (-5.715, 39.1886) -> (-5.715, 45.72)
  line L68 (-5.715, 45.72) -> (-2.54, 45.72)
  line L69 (-2.54, 45.72) -> (-2.54, 95.4786)
  line L70 (-2.54, 95.4786) -> (-113.665, 95.4786)
  line L71 (-113.665, 95.4786) -> (-113.665, 73.1704)
  line L72 (-59.69, 0) -> (-59.69, 6.5314)
  line L73 (-59.69, 6.5314) -> (-56.515, 6.5314)
  line L74 (-56.515, 6.5314) -> (-56.515, 0)
  line L75 (-56.515, 0) -> (-59.69, 0)
  line L76 (-59.69, 39.1886) -> (-56.515, 39.1886)
  line L77 (-56.515, 39.1886) -> (-56.515, 32.6571)
  line L78 (-56.515, 32.6571) -> (-59.69, 32.6571)
  line L79 (-59.69, 32.6571) -> (-59.69, 39.1886)
  line L80 (-59.69, 32.6571) -> (-56.515, 32.6571)
  line L81 (-56.515, 32.6571) -> (-56.515, 26.1257)
  line L82 (-56.515, 26.1257) -> (-59.69, 26.1257)
  line L83 (-59.69, 26.1257) -> (-59.69, 32.6571)
  line L84 (-59.69, 26.1257) -> (-56.515, 26.1257)
  line L85 (-56.515, 26.1257) -> (-56.515, 19.5943)
  line L86 (-56.515, 19.5943) -> (-59.69, 19.5943)
  line L87 (-59.69, 19.5943) -> (-59.69, 26.1257)
  line L88 (-56.515, 52.2514) -> (-56.515, 58.7829)
  line L89 (-59.69, 58.7829) -> (-59.69, 52.2514)
  line L90 (-56.515, 58.7829) -> (-59.69, 58.7829)
  line L91 (-59.69, 52.2514) -> (-56.515, 52.2514)
  line L92 (-59.69, 65.3143) -> (-59.69, 58.7829)
  line L93 (-56.515, 58.7829) -> (-56.515, 65.3143)
  line L94 (-59.69, 71.8457) -> (-59.69, 65.3143)
  line L95 (-56.515, 65.3143) -> (-59.69, 65.3143)
  line L96 (-56.515, 65.3143) -> (-56.515, 71.8457)
  line L97 (-56.515, 71.8457) -> (-59.69, 71.8457)
extrude "Extrude17" cut sketch "Sketch14" against normal blind 3.175 contours L88 L89 L90 L91 | L94 L95 L96 L97 bodies 3 in component "battery_box"
copy_body "CopyPasteBodies6" bodies 22 makes body 26 in component "battery_box"
move_body "Move9" bodies 26 to x (1, 0, 0) y (0, 1, 0) z (0, 0, 1) at (-137.16, 0, 0) in component "battery_box"
move_body "Align5" bodies 26 to x (1, 0, 0) y (0, 1, 0) z (0, 0, 1) at (83.185, 0, 0) in component "battery_box"
copy_body "CopyPasteBodies7" bodies 22 makes body 27 in component "battery_box"
move_body "Move10" bodies 27 to x (1, 0, 0) y (0, 1, 0) z (0, 0, 1) at (-160.02, 0, 0) in component "battery_box"
extrude "Extrude18" add 3 faces at (-47.4133, 23.3873, 22.0375) (-48.4717, 30.4822, 23.6751) (-48.4717, 38.5739, 25.5427) along direction (0, -0.224893, 0.974384) blind 3.81 on bodies 27 bodies 27 in component "battery_box"
move_body "Align6" bodies 27 to x (1, 0, 0) y (0, 1, 0) z (0, 0, 1) at (52.07, 0, 0) in component "battery_box"
combine "Combine20" operation cut target body 3 tool bodies 27 keep tools in component "battery_box"
combine "Combine21" operation cut target body 27 tool bodies 20 keep tools in component "battery_box"
combine "Combine22" operation cut target body 3 tool bodies 26 keep tools in component "battery_box"
combine "Combine23" operation cut target body 26 tool bodies 21 20 keep tools in component "battery_box"
combine "Combine24" operation cut target body 22 tool bodies 21 keep tools in component "battery_box"
extrude "Extrude19" add 1 faces at (57.5733, 0, 4.6567) along direction (0, 1, 0) blind 7.62 separate body on bodies 3 makes body 28 in component "battery_box"
combine "Combine25" operation add target body 3 tool bodies 28 keep tools in component "battery_box"
delete_body "RemoveBody6" bodies 28 in component "battery_box"
combine "Combine26" operation cut target body 26 tool bodies 3 keep tools in component "battery_box"
extrude "Extrude20" cut 1 faces at (58.6317, 3.81, 52.4933) along direction (0, -1, 0) blind 5.08 on bodies 26 bodies 26 in component "battery_box"
fillet "Fillet1" radius 8.89 2 edges at (2.54, 95.4786, 4.1275) (113.665, 95.4786, 4.1275) on bodies 3 in component "battery_box"
extrude "Extrude21" cut 1 faces at (42.545, 95.4786, 3.5983) along direction (0, -1, 0) blind 15.24 on bodies 3 bodies 3 in component "battery_box"
sketch "Sketch15" plane through (0, 0, 2.54) normal (0, 0, -1) x (-1, 0, 0) in component "battery_box"
  line L0 (-104.775, 80.2386) -> (-104.775, 95.4786)
  arc A0 (-104.775, 95.4786) -> (-113.665, 86.5886) centre (-104.775, 86.5886) ccw
  line L1 (-113.665, 86.5886) -> (-113.665, 73.1704)
  line L2 (-113.665, 73.1704) -> (-110.49, 73.1704)
  line L3 (-110.49, 73.1704) -> (-110.49, 65.3143)
  line L4 (-110.49, 65.3143) -> (-113.665, 65.3143)
  line L5 (-113.665, 65.3143) -> (-113.665, 58.7829)
  line L6 (-113.665, 58.7829) -> (-110.49, 58.7829)
  line L7 (-110.49, 58.7829) -> (-110.49, 52.2514)
  line L8 (-110.49, 52.2514) -> (-113.665, 52.2514)
  line L9 (-113.665, 52.2514) -> (-113.665, 45.72)
  line L10 (-113.665, 45.72) -> (-110.49, 45.72)
  line L11 (-110.49, 45.72) -> (-110.49, 39.1886)
  line L12 (-110.49, 39.1886) -> (-113.665, 39.1886)
  line L13 (-113.665, 39.1886) -> (-113.665, 32.6571)
  line L14 (-113.665, 32.6571) -> (-110.49, 32.6571)
  line L15 (-110.49, 32.6571) -> (-110.49, 26.1257)
  line L16 (-110.49, 26.1257) -> (-113.665, 26.1257)
  line L17 (-113.665, 26.1257) -> (-113.665, 19.5943)
  line L18 (-113.665, 19.5943) -> (-110.49, 19.5943)
  line L19 (-110.49, 19.5943) -> (-110.49, 13.0629)
  line L20 (-110.49, 13.0629) -> (-113.665, 13.0629)
  line L21 (-113.665, 13.0629) -> (-113.665, 6.5314)
  line L22 (-113.665, 6.5314) -> (-110.49, 6.5314)
  line L23 (-110.49, 6.5314) -> (-110.49, 0)
  line L24 (-110.49, 0) -> (-113.665, 0)
  line L25 (-113.665, 0) -> (-113.665, -3.175)
  line L26 (-113.665, -3.175) -> (-98.8483, -3.175)
  line L27 (-98.8483, -3.175) -> (-98.8483, 0)
  line L28 (-98.8483, 0) -> (-87.2067, 0)
  line L29 (-87.2067, 0) -> (-87.2067, -3.175)
  line L30 (-87.2067, -3.175) -> (-75.565, -3.175)
  line L31 (-75.565, -3.175) -> (-75.565, 0)
  line L32 (-75.565, 0) -> (-63.9233, 0)
  line L33 (-63.9233, 0) -> (-63.9233, -3.175)
  line L34 (-63.9233, -3.175) -> (-52.2817, -3.175)
  line L35 (-52.2817, -3.175) -> (-52.2817, 0)
  line L36 (-52.2817, 0) -> (-40.64, 0)
  line L37 (-40.64, 0) -> (-40.64, -3.175)
  line L38 (-40.64, -3.175) -> (-28.9983, -3.175)
  line L39 (-28.9983, -3.175) -> (-28.9983, 0)
  line L40 (-28.9983, 0) -> (-17.3567, 0)
  line L41 (-17.3567, 0) -> (-17.3567, -3.175)
  line L42 (-17.3567, -3.175) -> (-2.54, -3.175)
  line L43 (-2.54, -3.175) -> (-2.54, 0)
  line L44 (-2.54, 0) -> (-5.715, 0)
  line L45 (-5.715, 0) -> (-5.715, 6.5314)
  line L46 (-5.715, 6.5314) -> (-2.54, 6.5314)
  line L47 (-2.54, 6.5314) -> (-2.54, 13.0629)
  line L48 (-2.54, 13.0629) -> (-5.715, 13.0629)
  line L49 (-5.715, 13.0629) -> (-5.715, 19.5943)
  line L50 (-5.715, 19.5943) -> (-2.54, 19.5943)
  line L51 (-2.54, 19.5943) -> (-2.54, 26.1257)
  line L52 (-2.54, 26.1257) -> (-5.715, 26.1257)
  line L53 (-5.715, 26.1257) -> (-5.715, 32.6571)
  line L54 (-5.715, 32.6571) -> (-2.54, 32.6571)
  line L55 (-2.54, 32.6571) -> (-2.54, 39.1886)
  line L56 (-2.54, 39.1886) -> (-5.715, 39.1886)
  line L57 (-5.715, 39.1886) -> (-5.715, 45.72)
  line L58 (-5.715, 45.72) -> (-2.54, 45.72)
  line L59 (-2.54, 45.72) -> (-2.54, 52.2514)
  line L60 (-2.54, 52.2514) -> (-5.715, 52.2514)
  line L61 (-5.715, 52.2514) -> (-5.715, 58.7829)
  line L62 (-5.715, 58.7829) -> (-2.54, 58.7829)
  line L63 (-2.54, 58.7829) -> (-2.54, 65.3143)
  line L64 (-2.54, 65.3143) -> (-5.715, 65.3143)
  line L65 (-5.715, 65.3143) -> (-5.715, 73.1704)
  line L66 (-5.715, 73.1704) -> (-2.54, 73.1704)
  line L67 (-2.54, 73.1704) -> (-2.54, 86.5886)
  arc A1 (-2.54, 86.5886) -> (-11.43, 95.4786) centre (-11.43, 86.5886) ccw
  line L68 (-11.43, 95.4786) -> (-11.43, 80.2386)
  line L69 (-11.43, 80.2386) -> (-104.775, 80.2386)
  line L70 (-56.515, 58.7829) -> (-56.515, 52.2514)
  line L71 (-56.515, 52.2514) -> (-59.69, 52.2514)
  line L72 (-59.69, 52.2514) -> (-59.69, 58.7829)
  line L73 (-59.69, 58.7829) -> (-56.515, 58.7829)
  line L74 (-59.69, 65.3143) -> (-59.69, 73.1704)
  line L75 (-59.69, 73.1704) -> (-56.515, 73.1704)
  line L76 (-56.515, 73.1704) -> (-56.515, 65.3143)
  line L77 (-56.515, 65.3143) -> (-59.69, 65.3143)
  line L78 (-59.69, 19.5943) -> (-56.515, 19.5943)
  line L79 (-56.515, 19.5943) -> (-56.515, 13.0629)
  line L80 (-56.515, 13.0629) -> (-59.69, 13.0629)
  line L81 (-59.69, 13.0629) -> (-59.69, 19.5943)
  line L82 (-59.69, 32.6571) -> (-56.515, 32.6571)
  line L83 (-56.515, 32.6571) -> (-56.515, 26.1257)
  line L84 (-56.515, 26.1257) -> (-59.69, 26.1257)
  line L85 (-59.69, 26.1257) -> (-59.69, 32.6571)
  line L86 (-59.69, 45.72) -> (-56.515, 45.72)
  line L87 (-56.515, 45.72) -> (-56.515, 39.1886)
  line L88 (-56.515, 39.1886) -> (-59.69, 39.1886)
  line L89 (-59.69, 39.1886) -> (-59.69, 45.72)
  line L90 (-113.665, 79.8795) -> (-2.54, 79.8795)
  line L91 (-2.54, 79.8795) -> (-2.54, 99.06)
  line L92 (-2.54, 99.06) -> (-113.665, 99.06)
  line L93 (-113.665, 99.06) -> (-113.665, 79.8795)
extrude "Extrude22" cut sketch "Sketch15" against normal blind 5.08 contours L0 A0 L1 L67 A1 L68 L69 L90 L91 L93 bodies 3 in component "battery_box"
fillet "Fillet2" radius 5.08 2 edges at (2.54, 79.8795, 4.1275) (113.665, 79.8795, 4.1275) on bodies 3 in component "battery_box"
component "BatteryTower" placed x (1, 0, 0) y (0, 1, 0) z (0, 0, 1) at (0, 0, 0)
component "battery_box" placed x (1, 0, 0) y (0, 1, 0) z (0, 0, 1) at (-0.608, -1.4847, -1.7266) in component "BatteryTower"
equation "bd = 0.6 in" comment "Battery Diameter"
equation "bl = 2 in" comment "Battery Length"
equation "t = 0.125 in" comment "Material Thickness"
equation "d4 = ( t * 2 ) + ( bd * 3 )"
equation "d5 = ( bl * 2 ) + ( t * 3 )"
equation "d6 = t"
equation "d9 = t"
equation "d11 = t"
equation "d13 = t"
equation "d16 = t"
equation "d18 = t"
equation "d19 = bd"
equation "d26 = -t"